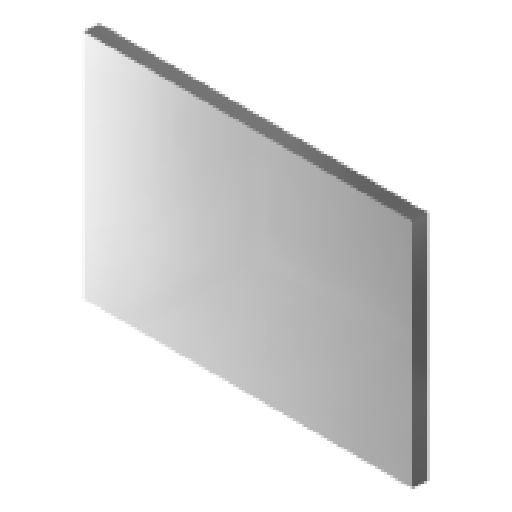
# Autodesk Inventor part: 00_3M_StickyPad
Saved by Autodesk Inventor 2025.1 (Build 291241000, 241)
## iProperties
Created: 2024-10-22
Part Number: 00_3M_StickyPad
Material: Generic
Document SubType Name: Modeling
Designer: Muriel
Density: 1 g/cm^3
Appearance: Chrome - Polished
Author: Muriel
Autodesk Inventor part; units mm, degrees
ref_plane "YZ Plane" through (0, 0, 0) normal (1, 0, 0) x (0, 1, 0)
ref_plane "XZ Plane" through (0, 0, 0) normal (0, 1, 0) x (-1, 0, 0)
ref_plane "XY Plane" through (0, 0, 0) normal (0, 0, 1) x (1, 0, 0)
sketch "Sketch1" plane through (0, 0, 0) normal (0, 0, 1) x (1, 0, 0)
  line L0 (-11, -7.75) -> (11, -7.75)
  line L1 (11, -7.75) -> (11, 7.75)
  line L2 (11, 7.75) -> (-11, 7.75)
  line L3 (-11, 7.75) -> (-11, -7.75)
  line L4 (-11, -7.75) -> (11, 7.75) construction
  line L5 (11, -7.75) -> (-11, 7.75) construction
  point P0 (0, 0)
  dimension "d0" = 22
  dimension "d1" = 15.5
  constraints: 12 end point, 2 midpoint, 2 parallel, 1 horizontal, 1 perpendicular
  measures "d0" distance of L2.end L1.end
  measures "d1" distance of L1.end L0.end
extrude "Extrusion1" add sketch "Sketch1" along normal blind 1
body "Solid1"
